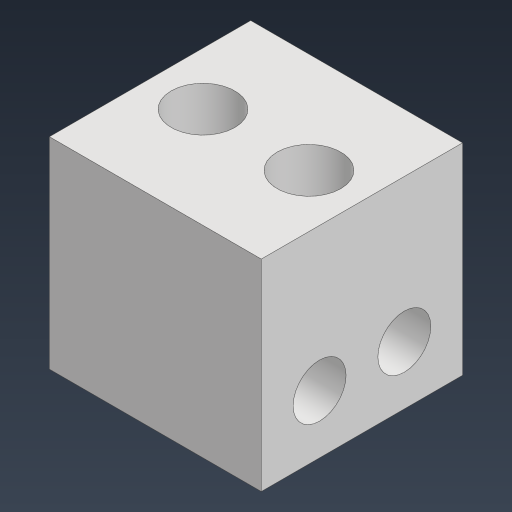
# Autodesk Inventor part: glue_test_PULLING
Saved by Autodesk Inventor 2023 (Build 270158000, 158)
## iProperties
Created: 2025-12-21
Part Number: glue_test_PULLING
Material: Generic
Document SubType Name: Modeling
Designer: szymo
Density: 1 g/cm^3
Appearance: Default
Author: szymo
Autodesk Inventor part; units mm, degrees
ref_plane "YZ Plane" through (0, 0, 0) normal (1, 0, 0) x (0, 1, 0)
ref_plane "XZ Plane" through (0, 0, 0) normal (0, 1, 0) x (-1, 0, 0)
ref_plane "XY Plane" through (0, 0, 0) normal (0, 0, 1) x (1, 0, 0)
sketch "Sketch1" plane through (0, 0, 0) normal (0, 1, 0) x (-1, 0, 0)
  line L0 (5, 4.75) -> (-5, 4.75)
  line L1 (-5, 4.75) -> (-5, -4.75)
  line L2 (-5, -4.75) -> (5, -4.75)
  line L3 (5, -4.75) -> (5, 4.75)
  line L4 (5, 4.75) -> (-5, -4.75) construction
  line L5 (-5, 4.75) -> (5, -4.75) construction
  circle A0 centre (-2.5, 0) radius 1.5
  circle A1 centre (2.5, 0) radius 1.5
  line L6 (-5, 0) -> (-2.5, 0) construction
  line L7 (-2.5, 0) -> (2.5, 0) construction
  line L8 (2.5, 0) -> (5.0355, 0) construction
  point P0 (0, 0)
  dimension "d0" = 10
  dimension "d1" = 9.5
  dimension "d2" = 3
  dimension "d3" = 3
  dimension "d4" = 2.5
  dimension "d5" = 2.5
  dimension "d6" = 2.5
  dimension "d7" = 2.5
  constraints: 18 end point, 3 horizontal, 3 midpoint, 2 centre point, 2 parallel, 1 perpendicular, 1 point on line
  measures "d0" distance of L2.end L1.end
  measures "d1" distance of L1.end L0.end
  measures "d2" diameter of A0
  measures "d3" diameter of A1
  measures "d4" distance of L6.end point (0, 0)
  measures "d5" distance of point (0, 0) L7.end
  measures "d6" distance from line of L1 L6.end
  measures "d7" distance from line of L3 L7.end
extrude "Extrusion1" add sketch "Sketch1" along normal blind 9.5
extrude "Extrusion2" add sketch "Sketch1" along normal blind 5.5 contours A0 | A1
sketch "Sketch2" plane through (5, 0, 4.75) normal (1, 0, 0) x (0, 0, -1)
  line L0 (0, 0) -> (9.5, 0) projected
  line L1 (9.5, 0) -> (9.5, 9.5) projected
  line L2 (0, 9.5) -> (9.5, 9.5) projected
  line L3 (0, 0) -> (0, 9.5) projected
  circle A0 centre (2.75, 2.75) radius 1.25
  circle A1 centre (6.75, 2.75) radius 1.25
  point P0 (4.75, 0)
  dimension "d12" = 2.5
  dimension "d13" = 2.5
  dimension "d14" = 2.75
  dimension "d15" = 2.75
  dimension "d16" = 2.75
  dimension "d17" = 2.75
  constraints: 2 centre point
  measures "d12" diameter of A0
  measures "d13" diameter of A1
  measures "d14" distance from line of L3 A0.centre
  measures "d15" distance from line of L1 A1.centre
  measures "d16" distance from line of L0 A1.centre
  measures "d17" distance from line of L0 A0.centre
extrude "Extrusion3" cut sketch "Sketch2" against normal through all contours A0 | A1
equation "\"d3\" = d2"
equation "\"d5\" = d4"
equation "\"d6\" = d4"
body "Solid1"
